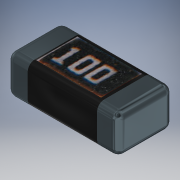
# Autodesk Inventor part: 603_Resistor
Saved by Autodesk Inventor 2017 SP1 (Build 210196100, 196)
## iProperties
Created: 2016-08-28
Part Number: 603_Resistor
Material: Generic
Document SubType Name: Modeling
Designer: jwrjc
Density: 1 g/cm^3
Appearance: Default
Author: jwrjc
Autodesk Inventor part; units mm, degrees
ref_plane "YZ Plane" through (0, 0, 0) normal (1, 0, 0) x (0, 1, 0)
ref_plane "XZ Plane" through (0, 0, 0) normal (0, 1, 0) x (-1, 0, 0)
ref_plane "XY Plane" through (0, 0, 0) normal (0, 0, 1) x (1, 0, 0)
sketch "Sketch1" plane through (0, 0, 0) normal (0, 0, 1) x (1, 0, 0)
  line L0 (0.4074, 0.3156) -> (-0.5726, 0.3156)
  line L1 (-0.5726, 0.3156) -> (-0.5726, -0.4644)
  line L2 (-0.5726, -0.4644) -> (0.4074, -0.4644)
  line L3 (0.4074, -0.4644) -> (0.4074, 0.3156)
  line L4 (0.4074, 0.3156) -> (0.7074, 0.3156)
  line L5 (0.7074, 0.3156) -> (0.7074, -0.4644)
  line L6 (0.7074, -0.4644) -> (0.4074, -0.4644)
  line L7 (0.4074, -0.4644) -> (0.4074, 0.3156)
  line L8 (-0.5726, 0.3156) -> (-0.8726, 0.3156)
  line L9 (-0.8726, 0.3156) -> (-0.8726, -0.4644)
  line L10 (-0.8726, -0.4644) -> (-0.5726, -0.4644)
  line L11 (-0.5726, -0.4644) -> (-0.5726, 0.3156)
  line L12 (-0.5122, 0.1851) -> (0.3336, 0.1851)
  line L13 (0.3336, 0.1851) -> (0.3336, -0.3622) construction
  line L14 (0.3336, -0.3622) -> (-0.5122, -0.3622) construction
  line L15 (-0.5122, -0.3622) -> (-0.5122, 0.1851) construction
  point P0 (0, 0)
  dimension "d8" = 0.3
  dimension "d13" = 0.3
  dimension "d15" = 0.98
  dimension "d16" = 0.78
  dimension "d41" = 0.0738
  dimension "d43" = 0.1022
  dimension "d48" = 0.1305
  constraints: 24 end point, 6 parallel, 3 horizontal, 3 perpendicular, 2 point on line, 2 other
  measures "d8" distance of L5.end L6.end
  measures "d13" distance of L9.end L10.end
  measures "d15" distance of L0.start L0.end
  measures "d16" distance of L4.end L5.end
  measures "d41" distance between parallel lines of L13 L3
  measures "d43" distance between parallel lines of L2 L14
  measures "d48" distance between parallel lines of L0 L12
extrude "Extrusion1" add sketch "Sketch1" along normal blind 0.55 contours L3 L2 L1 L0
extrude "Extrusion2" add sketch "Sketch1" along normal blind 0.55 separate body contours L4 L5 L6 L3 | L1 L10 L9 L8
sketch "Sketch2" plane through (0, 0, 0.55) normal (0, 0, 1) x (1, 0, 0)
  line L0 (-0.5533, 0.2245) -> (0.3669, 0.2245) construction
  line L1 (0.3669, 0.2245) -> (0.3669, -0.3709) construction
  line L2 (0.3669, -0.3709) -> (-0.5533, -0.3709) construction
  line L3 (-0.5533, -0.3709) -> (-0.5533, 0.2245) construction
  line L4 (0.4074, 0.3156) -> (-0.5726, 0.3156) projected
  line L5 (-0.5726, 0.3156) -> (-0.5726, -0.4644) projected
  line L6 (-0.5726, -0.4644) -> (0.4074, -0.4644) projected
  line L7 (0.4074, -0.4644) -> (0.4074, 0.3156) projected
  point P0 (0, 0)
  constraints: 2 other
decal "Decal1"
fillet "Fillet1" radius 0.1 20 edges at (-0.0826, -0.4644, 0.55) (-0.0826, 0.3156, 0.55) (-0.0826, -0.4644, 0) (-0.0826, 0.3156, 0) (0.7074, -0.0744, 0.55) (0.5574, -0.4644, 0.55) (-0.7226, -0.4644, 0.55) (-0.8726, -0.0744, 0.55) (-0.7226, 0.3156, 0.55) (0.5574, 0.3156, 0.55) (0.7074, -0.4644, 0.275) (0.5574, -0.4644, 0) (-0.7226, -0.4644, 0) (-0.8726, -0.0744, 0) (-0.8726, -0.4644, 0.275) (-0.8726, 0.3156, 0.275) (-0.7226, 0.3156, 0) (0.5574, 0.3156, 0) (0.7074, 0.3156, 0.275) (0.7074, -0.0744, 0)
body "Solid1"
body "Solid2"
